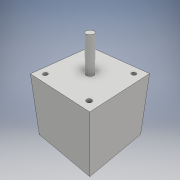
# Autodesk Inventor part: Motor nema
Saved by Autodesk Inventor 2018 (Build 220112000, 112)
## iProperties
Created: 2019-11-10
Part Number: Motor nema
Material: Типовые
Document SubType Name: Modeling
Designer: cosko
Density: 1 g/cm^3
Appearance: По умолчанию
Mass: 73.8616 g
Surface Area: 125.068 cm^2
Volume: 73.8616 cm^3
Author: cosko
Autodesk Inventor part; units mm, degrees
ref_plane "YZ Plane" through (0, 0, 0) normal (1, 0, 0) x (0, 1, 0)
ref_plane "XZ Plane" through (0, 0, 0) normal (0, 1, 0) x (-1, 0, 0)
ref_plane "XY Plane" through (0, 0, 0) normal (0, 0, 1) x (1, 0, 0)
sketch "Эскиз1" plane through (0, 0, 0) normal (0, 0, 1) x (1, 0, 0)
  line L0 (-21, -21.15) -> (21, -21.15)
  line L1 (21, -21.15) -> (21, 21.15)
  line L2 (21, 21.15) -> (-21, 21.15)
  line L3 (-21, 21.15) -> (-21, -21.15)
  line L4 (-21, -21.15) -> (21, 21.15) construction
  line L5 (21, -21.15) -> (-21, 21.15) construction
  line L6 (-21, 0) -> (21, 0)
  line L7 (0, 21.15) -> (0, -21.15)
  line L8 (21, 0) -> (21, 15.5) construction
  line L9 (21, 0) -> (21, -16) construction
  line L10 (21, -16) -> (-21, -16) construction
  line L11 (21, 15.5) -> (-21, 15.5) construction
  line L12 (0, 21.15) -> (-15.5, 21.15) construction
  line L13 (0, 21.15) -> (15.5, 21.15) construction
  line L14 (15.5, 21.15) -> (15.5, -21.15) construction
  line L15 (-15.5, 21.15) -> (-15.5, -21.15) construction
  circle A0 centre (-15.5, 15.5) radius 1.5
  circle A1 centre (15.5, 15.5) radius 1.5
  circle A2 centre (15.5, -16) radius 1.5
  circle A3 centre (-15.5, -16) radius 1.5
  circle A4 centre (0, 0) radius 2.5
  dimension "d0" = 42
  dimension "d1" = 42.3
  dimension "d2" = 15.5
  dimension "d3" = 16
  dimension "d4" = 15.5
  dimension "d5" = 15.5
  dimension "d6" = 3
  dimension "d7" = 3
  dimension "d8" = 3
  dimension "d9" = 3
  dimension "d10" = 5
  constraints: 32 end point, 16 point on line, 6 midpoint, 5 centre point, 5 perpendicular, 2 parallel, 1 coincident, 1 horizontal
  measures "d0" distance of L2.end L1.end
  measures "d1" distance of L1.end L0.end
  measures "d2" distance of L6.end L8.end
  measures "d3" distance of L6.end L9.end
  measures "d4" distance of L7.start L12.end
  measures "d5" distance of L7.start L13.end
  measures "d6" diameter of A0
  measures "d7" diameter of A1
  measures "d8" diameter of A2
  measures "d9" diameter of A3
  measures "d10" diameter of A4
extrude "Выдавливание1" add sketch "Эскиз1" against normal blind 42
extrude "Выдавливание2" add sketch "Эскиз1" along normal blind 22 contours A4 L6 L7 | L7 L6 A4 | A4 L7 L6 | L7 A4 L6
